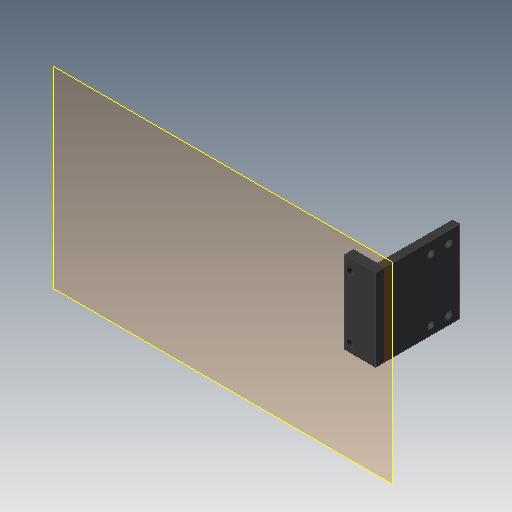
# Autodesk Inventor part: cellSTORM_Laserrotator_v0
Saved by Autodesk Inventor 2019.4 (Build 234330000, 330)
## iProperties
Created: 2020-07-31
Part Number: cellSTORM_Laserrotator_v0
Material: Generic
Document SubType Name: Modeling
Designer: diederichbenedict
Density: 1 g/cm^3
Appearance: Default
Author: diederichbenedict
Autodesk Inventor part; units mm, degrees
ref_plane "YZ Plane" through (0, 0, 0) normal (1, 0, 0) x (0, 1, 0)
ref_plane "XZ Plane" through (0, 0, 0) normal (0, 1, 0) x (-1, 0, 0)
ref_plane "XY Plane" through (0, 0, 0) normal (0, 0, 1) x (1, 0, 0)
ref_plane "Work Plane1" through (0, 0, 0) normal (0, 0, 1) x (1, 0, 0)
sketch "Sketch1" plane through (0, 0, 0) normal (0, 0, 1) x (1, 0, 0)
  line L0 (63.5, -8.73) -> (63.5, 39.27) projected
  line L1 (60.6576, -39.5) -> (69.5, -30.6576) projected
  line L2 (69.5, -30.6576) -> (69.5, 39.5) projected
  line L3 (69.5, 39.5) -> (1.55, 39.5) projected
  line L4 (1.55, 39.5) -> (-11.5, 34.5) projected
  line L5 (-11.5, 34.5) -> (-67.5, 34.5) projected
  line L6 (-67.5, 34.5) -> (-69.5, 32.5) projected
  line L7 (-69.5, 32.5) -> (-69.5, -23.5) projected
  line L8 (-69.5, -23.5) -> (-67.5, -25.5) projected
  line L9 (-67.5, -25.5) -> (-11.5, -25.5) projected
  line L10 (-11.5, -25.5) -> (50.5667, -25.5) projected
  line L11 (50.5667, -25.5) -> (50.5667, -39.5) projected
  line L12 (50.5667, -39.5) -> (60.6576, -39.5) projected
  circle A0 centre (61.5, -3.73) radius 1.6 projected
  circle A1 centre (61.5, 6.27) radius 1.6 projected
  circle A2 centre (61.5, 34.27) radius 1.6 projected
  circle A3 centre (45.5, 34.27) radius 1.6 projected
  circle A4 centre (45.5, 6.27) radius 1.6 projected
  circle A5 centre (45.5, -3.73) radius 1.6 projected
  circle A6 centre (24.65, 15.77) radius 1.6 projected
  circle A7 centre (8.35, 15.77) radius 1.6 projected
  circle A8 centre (-14.5, 4.5) radius 1.95 projected
  circle A9 centre (-39.5, 29.5) radius 1.95 projected
  circle A10 centre (-64.5, -20.5) radius 1.95 projected
  circle A11 centre (-14.5, 29.5) radius 1.95 projected
  circle A12 centre (-64.5, 29.5) radius 1.95 projected
  circle A13 centre (-14.5, -20.5) radius 1.95 projected
  circle A14 centre (-39.5, -20.5) radius 1.95 projected
  circle A15 centre (-64.5, 4.5) radius 1.95 projected
  circle A16 centre (-57, 22) radius 4 projected
  circle A17 centre (-22, -13) radius 4 projected
  circle A18 centre (-57, -13) radius 4 projected
  circle A19 centre (-22, 22) radius 4 projected
  line L13 (70.0555, 39.5) -> (59.0555, 39.5)
  line L14 (59.0555, 39.5) -> (59.0555, 2.5)
  line L15 (59.0555, 2.5) -> (70.0555, 2.5)
  line L16 (70.0555, 2.5) -> (70.0555, 39.5)
  line L17 (70.0555, 39.5) -> (73.0555, 39.5)
  line L18 (73.0555, 39.5) -> (73.0555, 2.5)
  line L19 (73.0555, 2.5) -> (70.0555, 2.5)
  line L20 (70.0555, 2.5) -> (70.0555, 39.5)
  point P0 (0, 0)
  dimension "d0" = 11
  dimension "d1" = 37
  dimension "d2" = 3
  constraints: 16 end point, 4 parallel, 2 horizontal, 2 perpendicular, 2 point on line
  measures "d0" distance of L15.end L14.end
  measures "d1" distance of L14.end L13.end
  measures "d2" distance of L18.end L19.end
extrude "Extrusion1" add sketch "Sketch1" along normal blind 4 contours L15 L14 L3 L2 | L2 L13 L16 L15 | L16 L17 L18 L19
sketch "Sketch2" plane through (73.0555, 2.5, 0) normal (1, 0, 0) x (0, 0, -1)
  circle A0 centre (29, 3.77) radius 1.4 projected
  circle A1 centre (37, 3.77) radius 1.4 projected
  circle A2 centre (21, 3.77) radius 1.4 projected
  circle A3 centre (29, 31.77) radius 1.4 projected
  circle A4 centre (37, 31.77) radius 1.4 projected
  circle A5 centre (21, 31.77) radius 1.4 projected
  circle A6 centre (37, -6.23) radius 1.4 projected
  circle A7 centre (29, -6.23) radius 1.4 projected
  circle A8 centre (21, -6.23) radius 1.4 projected
  line L0 (13, 36.77) -> (45, 36.77) projected
  line L1 (13, 36.77) -> (13, -11.23) projected
  line L2 (45, -11.23) -> (13, -11.23) projected
  line L3 (45, 36.77) -> (45, -11.23) projected
  line L4 (0, 37) -> (-4, 37) projected
  line L5 (-4, 37) -> (34, 37)
  line L6 (34, 37) -> (34, 0)
  line L7 (34, 0) -> (-4, 0)
  line L8 (-4, 0) -> (-4, 37)
  point P0 (0, -2.5)
  dimension "d5" = 38
  constraints: 8 end point, 2 parallel, 1 coincident, 1 horizontal, 1 perpendicular
  measures "d5" distance of L6.end L7.end
extrude "Extrusion2" add sketch "Sketch2" against normal blind 3.2 contours L1 L7 L8 L4 L5 L6 L0 | L0 L6 L7 L1
body "Solid1"
